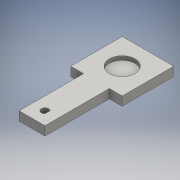
# Autodesk Inventor part: LowerArm
Saved by Autodesk Inventor 2016 (Build 200138000, 138)
## iProperties
Created: 2015-10-06
Part Number: LowerArm
Material: Generic
Document SubType Name: Modeling
Designer: alex
Density: 1 g/cm^3
Appearance: Default
Mass: 56.6565 g
Surface Area: 198.211 cm^2
Volume: 56.6565 cm^3
Author: alex
Autodesk Inventor part; units mm, degrees
ref_plane "YZ Plane" through (0, 0, 0) normal (1, 0, 0) x (0, 1, 0)
ref_plane "XZ Plane" through (0, 0, 0) normal (0, 1, 0) x (-1, 0, 0)
ref_plane "XY Plane" through (0, 0, 0) normal (0, 0, 1) x (1, 0, 0)
sketch "Sketch1" plane through (0, 0, 0) normal (0, 0, 1) x (1, 0, 0)
  line L0 (-20, 50) -> (20, 50)
  line L1 (20, 50) -> (20, 10)
  line L2 (-20, 10) -> (-20, 50)
  line L3 (-20, 10) -> (20, 10)
  line L4 (-10, 10) -> (10, 10)
  line L5 (10, 10) -> (10, -40)
  line L6 (10, -40) -> (-10, -40)
  line L7 (-10, -40) -> (-10, 10)
  point P0 (0, 0)
  dimension "d0" = 50
  dimension "d2" = 20
  dimension "d84" = 40
  dimension "d85" = 20
  dimension "d86" = 20
  dimension "d87" = 10
  dimension "d88" = 50
  constraints: 16 end point, 3 horizontal, 3 parallel, 2 perpendicular, 1 point on line
  measures "d0" distance from line of point (0, 0) L0
  measures "d2" distance from line of point (0, 0) L2
  measures "d84" distance between parallel lines of L0 L3
  measures "d85" distance from line of point (0, 0) L1
  measures "d86" distance between parallel lines of L5 L7
  measures "d87" distance from line of point (0, 0) L7
  measures "d88" distance between parallel lines of L3 L6
extrude "Extrusion11" add sketch "Sketch1" along normal blind 7
sketch "Sketch11" plane through (0, 0, 7) normal (0, 0, 1) x (1, 0, 0)
  circle A0 centre (0, 30) radius 10
  line L0 (20, 50) -> (-20, 50) projected
  line L1 (-20, 50) -> (-20, 10) projected
  point P0 (0, 0)
  point P1 (0, 50)
  point P2 (0, 50)
  point P3 (-20, 30)
  dimension "d91" = 20
  constraints: 3 midpoint, 1 centre point, 1 horizontal alignment, 1 vertical alignment
  measures "d91" diameter of A0
extrude "Extrusion12" cut sketch "Sketch11" against normal blind 3
sketch "Sketch12" plane through (0, 0, 7) normal (0, 0, 1) x (1, 0, 0)
  arc A0 (1.905, -27.9616) -> (1.905, -32.0384) centre (0, -30) ccw
  line L0 (-10, -40) -> (10, -40) projected
  line L1 (1.905, -27.9616) -> (1.905, -32.0384)
  point P0 (0, 0)
  point P1 (0, -40)
  dimension "d94" = 5.58
  dimension "d95" = 10
  dimension "d96" = 1.905
  constraints: 2 end point, 2 point on circle, 1 centre point, 1 midpoint, 1 vertical, 1 vertical alignment
  measures "d94" diameter of A0
  measures "d95" distance from line of L0 A0.centre
  measures "d96" distance from line of A0.centre L1
extrude "Extrusion13" cut sketch "Sketch12" against normal through all
body "Solid2"
